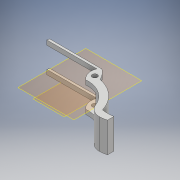
# Autodesk Inventor part: courbe
Saved by Autodesk Inventor 2017 (Build 210142000, 142)
## iProperties
Part Number: courbe
Material: Générique
Document SubType Name: Modeling
Designer: Thomas
Density: 1 g/cm^3
Appearance: Par défaut
Author: Thomas
Autodesk Inventor part; units mm, degrees
ref_plane "YZ Plane" through (0, 0, 0) normal (1, 0, 0) x (0, 1, 0)
ref_plane "XZ Plane" through (0, 0, 0) normal (0, 1, 0) x (-1, 0, 0)
ref_plane "XY Plane" through (0, 0, 0) normal (0, 0, 1) x (1, 0, 0)
ref_plane "Plan de construction1" through (0, 0, 0) normal (0, 0, 1) x (1, 0, 0)
sketch "Esquisse1" plane through (0, 0, 0) normal (0, 0, 1) x (1, 0, 0)
  arc A0 (39.951, -6.6629) -> (39.7815, -6.3404) centre (-6.5192, -30.8836) ccw
  arc A1 (37.1716, -5.7515) -> (36.5629, -4.7218) centre (-6.5192, -30.8836) ccw
  line L0 (-0.9849, 21.2268) -> (-0.9849, 19.2151)
  circle A2 centre (35, -6.3404) radius 2.25 projected
  circle A3 centre (35, -6.3404) radius 2.25
  line L1 (32.8713, 2.0538) -> (-13.1447, 2.0538)
  line L2 (-13.1447, 2.0538) -> (-13.6192, -0.0461)
  line L3 (-13.6192, -0.0461) -> (30.4775, -0.0461)
  arc A4 (31.5995, 2.0932) -> (31.5733, 2.0538) centre (41.1898, -4.3006) ccw
  arc A5 (30.4775, -0.0461) -> (33.9606, -13.278) centre (41.1898, -4.3006) ccw
  arc A6 (39.7815, -6.3404) -> (32.8713, 2.0538) centre (19.4137, -16.066) ccw
  arc A7 (67.9818, -35.5103) -> (74.3699, -34.5283) centre (66.006, -1.387) ccw
  line L4 (74.3699, -28.9007) -> (74.3699, -34.5283)
  arc A8 (64.3223, -28.9007) -> (39.951, -6.6629) centre (33.5629, -38.1376) ccw
  arc A9 (57.8312, -28.9007) -> (33.9606, -13.278) centre (35.6884, -36.6859) ccw
  arc A10 (57.8312, -28.9007) -> (70.9309, -35.2107) centre (68.2954, -23.9295) ccw
  arc A11 (39.951, -6.6629) -> (39.977, -6.7609) centre (69.3461, 1.0787) ccw
  arc A12 (64.3223, -28.9007) -> (74.3699, -28.9007) centre (69.3461, 1.0787) ccw
  point P0 (0, 0)
  point P1 (32.8713, 3.678)
  constraints: 27 point on circle, 12 centre point, 10 end point, 2 vertical, 1 coincident, 1 concentric, 1 parallel, 1 point on line
extrude "Extrusion1" add sketch "Esquisse1" along normal blind 4 contours A8 A12 L4 A7 A10 A9 A5 L3 L2 L1 A6 A0
ref_plane "Plan de construction2" through (0, 0, 13.25) normal (0, 0, 1) x (1, 0, 0)
mirror "Symétrie1" about plane through (0, 0, 13.25) normal (0, 0, 1) of "Extrusion1"
sketch "Esquisse4" plane through (0, 0, 4) normal (0, 0, 1) x (1, 0, 0)
  arc A0 (64.3223, -28.9007) -> (74.3699, -28.9007) centre (69.3461, 1.0787) ccw projected
  line L0 (74.3699, -34.5283) -> (74.3699, -28.9007) projected
  arc A1 (67.9818, -35.5103) -> (74.3699, -34.5283) centre (66.006, -1.387) ccw projected
  arc A2 (57.8312, -28.9007) -> (67.9818, -35.5103) centre (68.2954, -23.9295) ccw projected
  arc A3 (57.8312, -28.9007) -> (33.9606, -13.278) centre (35.6884, -36.6859) ccw projected
  arc A4 (64.3223, -28.9007) -> (39.951, -6.6629) centre (33.5629, -38.1376) ccw projected
  arc A5 (64.3223, -28.9007) -> (39.951, -6.6629) centre (33.5629, -38.1376) ccw projected
  line L1 (47.1623, -9.0426) -> (44.7261, -15.0241)
  arc A6 (57.8312, -28.9007) -> (33.9606, -13.278) centre (35.6884, -36.6859) ccw projected
  point P0 (0, 0)
  constraints: 4 point on circle, 2 end point
extrude "Extrusion5" add sketch "Esquisse4" along normal blind 19.25
